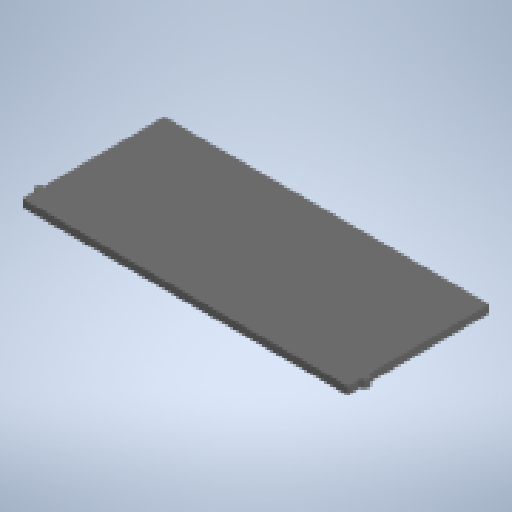
# Autodesk Inventor part: battery_case_cover
Saved by Autodesk Inventor 2024.1 (Build 281209000, 209)
## iProperties
Created: 2025-04-23
Part Number: battery_case_cover
Material: 一般
Document SubType Name: Modeling
Designer: hibik
Density: 1 g/cm^3
Appearance: 既定
Author: hibik
Autodesk Inventor part; units mm, degrees
ref_plane "YZ Plane" through (0, 0, 0) normal (1, 0, 0) x (0, 1, 0)
ref_plane "XZ Plane" through (0, 0, 0) normal (0, 1, 0) x (-1, 0, 0)
ref_plane "XY Plane" through (0, 0, 0) normal (0, 0, 1) x (1, 0, 0)
sketch "スケッチ1" plane through (0, 0, 0) normal (0, 1, 0) x (-1, 0, 0)
  line L0 (0, 0) -> (41.7, 0)
  line L1 (41.7, 0) -> (41.7, -18.2)
  line L2 (41.7, -18.2) -> (0, -18.2)
  line L3 (0, -18.2) -> (0, 0)
  dimension "d0" = 41.7
  dimension "d1" = 18.2
  constraints: 8 end point, 2 parallel, 1 horizontal, 1 perpendicular
  measures "d0" distance of L1.end L2.end
  measures "d1" distance of L0.end L1.end
extrude "押し出し1" add sketch "スケッチ1" along normal blind 1
sketch "スケッチ2" plane through (0, 0, 0) normal (0, -1, 0) x (1, 0, 0)
  line L0 (0, 0) -> (0, -18.2) projected
  circle A0 centre (0, -2.2) radius 0.55
  line L1 (-41.7, -18.2) -> (-41.7, 0) projected
  circle A1 centre (-41.7, -2.2) radius 0.55
  line L2 (-41.7, 0) -> (0, 0) projected
  dimension "d4" = 1.1
  dimension "d5" = 1.1
  dimension "d6" = 2.2
  constraints: 2 centre point, 2 point on line, 1 horizontal alignment
  measures "d4" diameter of A0
  measures "d5" diameter of A1
  measures "d6" distance from line of L2 A0.centre
extrude "押し出し2" add sketch "スケッチ2" against normal up to surface (1 mm away)
